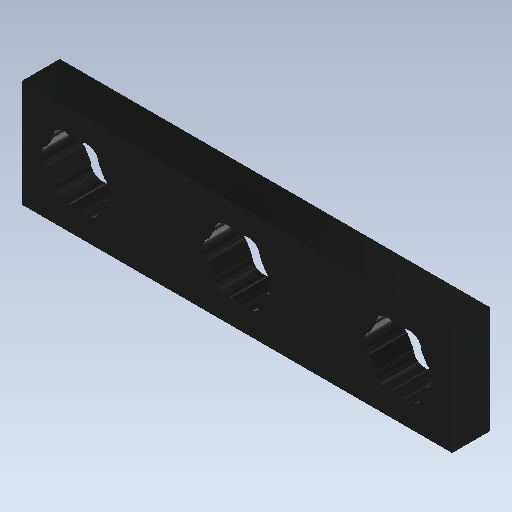
# Autodesk Inventor part: 胴体_サブフレーム_1_2
Saved by Autodesk Inventor 2020.4 (Build 244396000, 396)
## iProperties
Created: 2016-05-07
Part Number: 胴体_サブフレーム_1_2
Material: アセタール樹脂、黒
Document SubType Name: Modeling
Designer: hiroaki
Density: 1.425 g/cm^3
Appearance: 滑らか - 黒
Mass: 1.36213 g
Surface Area: 10.7398 cm^2
Volume: 0.955879 cm^3
Category: 胴体
Author: hiroaki
Autodesk Inventor part; units mm, degrees
ref_plane "YZ Plane" through (0, 0, 0) normal (1, 0, 0) x (0, 1, 0)
ref_plane "XZ Plane" through (0, 0, 0) normal (0, 1, 0) x (-1, 0, 0)
ref_plane "XY Plane" through (0, 0, 0) normal (0, 0, 1) x (1, 0, 0)
sketch "スケッチ1" plane through (0, 0, 0) normal (0, 0, 1) x (1, 0, 0)
  line L0 (-20, -5) -> (20, -5)
  line L1 (20, -5) -> (20, 5)
  line L2 (20, 5) -> (-20, 5)
  line L3 (-20, 5) -> (-20, -5)
  line L4 (-20, -5) -> (20, 5) construction
  line L5 (20, -5) -> (-20, 5) construction
  circle A0 centre (-15, 0) radius 1.55
  circle A1 centre (0, 0) radius 1.55
  line L6 (0, 0) -> (0, 5) construction
  line L7 (-12.5995, 5) -> (4.4005, 5) construction
  line L8 (-8.5, -4) -> (8.5, -4) construction
  line L9 (-13.4065, -2.76) -> (-16.5935, -2.76)
  line L10 (-16.5935, -2.76) -> (-18.187, 0)
  line L11 (-18.187, 0) -> (-16.5935, 2.76)
  line L12 (-16.5935, 2.76) -> (-13.4065, 2.76)
  line L13 (-13.4065, 2.76) -> (-11.813, 0)
  line L14 (-11.813, 0) -> (-13.4065, -2.76)
  circle A2 centre (-17.137, 0) radius 1.05
  circle A3 centre (-16.0685, -1.8507) radius 1.05
  circle A4 centre (-13.9315, -1.8507) radius 1.05
  circle A5 centre (-12.863, 0) radius 1.05
  circle A6 centre (-13.9315, 1.8507) radius 1.05
  circle A7 centre (-16.0685, 1.8507) radius 1.05
  circle A8 centre (15, 0) radius 1.55
  line L15 (13.4065, -2.76) -> (16.5935, -2.76)
  line L16 (16.5935, -2.76) -> (18.187, 0)
  line L17 (18.187, 0) -> (16.5935, 2.76)
  line L18 (16.5935, 2.76) -> (13.4065, 2.76)
  line L19 (13.4065, 2.76) -> (11.813, 0)
  line L20 (11.813, 0) -> (13.4065, -2.76)
  circle A9 centre (17.137, 0) radius 1.05
  circle A10 centre (16.0685, -1.8507) radius 1.05
  circle A11 centre (13.9315, -1.8507) radius 1.05
  circle A12 centre (12.863, 0) radius 1.05
  circle A13 centre (13.9315, 1.8507) radius 1.05
  circle A14 centre (16.0685, 1.8507) radius 1.05
  circle A15 centre (-15, 0) radius 5 construction
  line L21 (1.5935, -2.76) -> (-1.5935, -2.76)
  line L22 (-1.5935, -2.76) -> (-3.187, 0)
  line L23 (-3.187, 0) -> (-1.5935, 2.76)
  line L24 (-1.5935, 2.76) -> (1.5935, 2.76)
  line L25 (1.5935, 2.76) -> (3.187, 0)
  line L26 (3.187, 0) -> (1.5935, -2.76)
  circle A16 centre (-2.137, 0) radius 1.05
  circle A17 centre (-1.0685, -1.8507) radius 1.05
  circle A18 centre (1.0685, -1.8507) radius 1.05
  circle A19 centre (2.137, 0) radius 1.05
  circle A20 centre (1.0685, 1.8507) radius 1.05
  circle A21 centre (-1.0685, 1.8507) radius 1.05
  point P0 (-16.5935, -2.76)
  point P1 (-13.4065, -2.76)
  point P2 (-11.813, 0)
  point P3 (-13.4065, 2.76)
  point P4 (-16.5935, 2.76)
  point P5 (16.5935, -2.76)
  point P6 (13.4065, -2.76)
  point P7 (11.813, 0)
  point P8 (13.4065, 2.76)
  point P9 (16.5935, 2.76)
  point P10 (-1.5935, -2.76)
  point P11 (1.5935, -2.76)
  point P12 (3.187, 0)
  point P13 (1.5935, 2.76)
  dimension "d19" = 2.1
  dimension "d1" = 3.1
  dimension "d4" = 15
  dimension "d5" = 10
  dimension "d20" = 5.52
  dimension "d23" = 360
  dimension "d33" = 360
  constraints: 54 end point, 19 symmetric about line, 9 horizontal alignment, 6 coincident, 6 vertical, 5 horizontal, 5 midpoint, 4 centre point, 2 collinear, 2 parallel, 2 tangent, 1 equal radius, 1 perpendicular, 113 other
  measures "d1" diameter of A0
  measures "d4" distance of point (0, 0) A0.centre
  measures "d5" distance of L2.end L0.start
  measures "d20" distance between parallel lines of L12 L9
extrude "押し出し1" add sketch "スケッチ1" along normal blind 3.5
